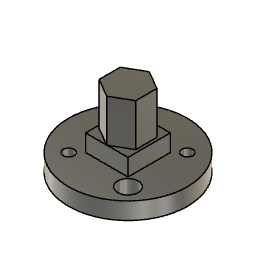
hex_peg_V2 v1 (Autodesk Fusion 360 design; units mm, degrees)
Autodesk Fusion 360 part; units mm, degrees
sketch "Sketch1" plane through (0, 0, 0) normal (0, 0, 1) x (1, 0, 0)
  line L0 (12.5, -12.5) -> (-12.5, -12.5)
  line L1 (-12.5, -12.5) -> (-12.5, 12.5)
  line L2 (-12.5, 12.5) -> (12.5, 12.5)
  line L3 (12.5, 12.5) -> (12.5, -12.5)
  line L4 (12.5, -12.5) -> (-12.5, 12.5) construction
  line L5 (-12.5, -12.5) -> (12.5, 12.5) construction
  dimension "d1" = 25
  dimension "d2" = 25
  constraint horizontal L0
  constraint perpendicular L0 L1
  constraint parallel L0 L2
  constraint parallel L1 L3
  constraint coincident L4 origin
  constraint coincident L5 origin
  measures "d1" distance of L1.end L2.end
  measures "d2" distance of L0.end L1.end
extrude "Extrude1" add sketch "Sketch1" along normal blind 10 makes body 1
sketch "Sketch4" plane through (0, 0, 0) normal (0, 0, 1) x (1, 0, 0)
  circle A0 centre (17.5, 17.5) radius 3.25
  circle A1 centre (-17.5, -17.5) radius 3.25
  circle A2 centre (-17.5, 17.5) radius 3.25
  circle A3 centre (17.5, -17.5) radius 3.25
  circle A4 centre (0, 0) radius 35
  circle A5 centre (-17.5, 17.5) radius 6
  circle A6 centre (17.5, -17.5) radius 6
  dimension "d15" = 360
  dimension "d16" = 70
  dimension "d17" = 17.5
  dimension "d18" = 17.5
  dimension "d19" = 6.5
  dimension "d20" = 12
  dimension "d21" = 12
  constraint coincident A4.centre origin
  constraint concentric A2 A5
  constraint concentric A3 A6
  measures "d16" diameter of A4
  measures "d17" vertical distance of A4.centre A0.centre
  measures "d18" horizontal distance of A4.centre A0.centre
  measures "d19" diameter of A0
  measures "d20" diameter of A5
  measures "d21" diameter of A6
extrude "Extrude4" add sketch "Sketch4" against normal blind 10 contours A4 bodies 1
sketch "Sketch5" plane through (0, 0, 10) normal (0, 0, 1) x (-1, 0, 0)
  circle A0 centre (0, 0) radius 12.5 construction
  line L0 (12.5, 12.5) -> (-12.5, 12.5)
  line L1 (0, 12.5) -> (-10.8253, 6.25)
  line L2 (-10.8253, 6.25) -> (-10.8253, -6.25)
  line L3 (-10.8253, -6.25) -> (0, -12.5)
  line L4 (0, -12.5) -> (10.8253, -6.25)
  line L5 (10.8253, -6.25) -> (10.8253, 6.25)
  line L6 (10.8253, 6.25) -> (0, 12.5)
  constraint coincident A0.centre origin
  constraint tangent A0 L0
  constraint midpoint L0 L1.start
extrude "Extrude5" add sketch "Sketch5" along normal blind 25 bodies 1
split "Split1" by plane through (0, 0, 0) normal (0, 0, 1) bodies 1 makes body 2 at (-3.6084, 2.0833, 35)
split "Split2" by plane through (0, 0, 10) normal (0, 0, 1) bodies 2 makes body 3 at (-3.6084, 2.0833, 35)
